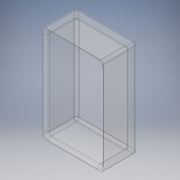
# Autodesk Inventor part: Outer Block
Saved by Autodesk Inventor 2017 (Build 210142000, 142)
## iProperties
Created: 2017-10-25
Part Number: Outer Block
Material: Polycarbonate, Clear
Document SubType Name: Modeling
Designer: Tripl_000
Density: 1.2 g/cm^3
Appearance: Polycarbonate - Clear
Author: Tripl_000
Autodesk Inventor part; units mm, degrees
ref_plane "YZ Plane" through (0, 0, 0) normal (1, 0, 0) x (0, 1, 0)
ref_plane "XZ Plane" through (0, 0, 0) normal (0, 1, 0) x (-1, 0, 0)
ref_plane "XY Plane" through (0, 0, 0) normal (0, 0, 1) x (1, 0, 0)
sketch "Sketch3" plane through (0, 0, 0) normal (0, 0, 1) x (1, 0, 0)
  line L0 (-20.25, 32.25) -> (20.25, 32.25)
  line L1 (20.25, 32.25) -> (20.25, -32.25)
  line L2 (20.25, -32.25) -> (-20.25, -32.25)
  line L3 (-20.25, -32.25) -> (-20.25, 32.25)
  line L4 (-20.25, 32.25) -> (20.25, -32.25) construction
  line L5 (20.25, 32.25) -> (-20.25, -32.25) construction
  point P0 (0, 0)
  dimension "d9" = 40.5
  dimension "d10" = 64.5
  constraints: 12 end point, 2 midpoint, 2 parallel, 1 horizontal, 1 perpendicular
  measures "d9" distance of L0.start L0.end
  measures "d10" distance of L2.end L0.start
extrude "Extrusion3" add sketch "Sketch3" along normal blind 22.5
sketch "Sketch4" plane through (0, 0, 22.5) normal (0, 0, 1) x (1, 0, 0)
  line L0 (-18, 30) -> (18, 30)
  line L1 (18, 30) -> (18, -30)
  line L2 (18, -30) -> (-18, -30)
  line L3 (-18, -30) -> (-18, 30)
  line L4 (-18, 30) -> (18, -30) construction
  line L5 (18, 30) -> (-18, -30) construction
  point P0 (0, 0)
  dimension "d13" = 36
  dimension "d14" = 60
  constraints: 12 end point, 2 midpoint, 2 parallel, 1 horizontal, 1 perpendicular
  measures "d13" distance of L0.start L0.end
  measures "d14" distance of L2.end L0.start
extrude "Extrusion4" cut sketch "Sketch4" against normal blind 20
fillet "Fillet2" radius 2 12 edges at (-18, -30, 12.5) (-18, 30, 12.5) (18, -30, 12.5) (18, 30, 12.5) (18, 0, 2.5) (0, 30, 2.5) (-18, 0, 2.5) (0, -30, 2.5) (0, -30, 22.5) (-18, 0, 22.5) (0, 30, 22.5) (18, 0, 22.5)
fillet "Fillet3" radius 1.5 8 edges at (20.25, 32.25, 11.25) (-20.25, 32.25, 11.25) (20.25, -32.25, 11.25) (-20.25, -32.25, 11.25) (20.25, 0, 0) (0, 32.25, 0) (-20.25, 0, 0) (0, -32.25, 0)
body "Solid2"
